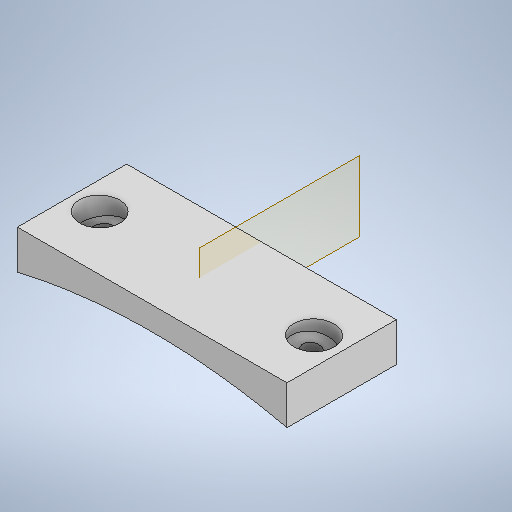
# Autodesk Inventor part: MountPlateV1
Saved by Autodesk Inventor 2025 (Build 290162000, 162)
## iProperties
Created: 2024-05-27
Part Number: MountPlateV1
Material: Generic
Document SubType Name: Modeling
Designer: mason
Density: 1 g/cm^3
Appearance: Default
Author: mason
Autodesk Inventor part; units mm, degrees
ref_plane "YZ Plane" through (0, 0, 0) normal (1, 0, 0) x (0, 1, 0)
ref_plane "XZ Plane" through (0, 0, 0) normal (0, 1, 0) x (-1, 0, 0)
ref_plane "XY Plane" through (0, 0, 0) normal (0, 0, 1) x (1, 0, 0)
sketch "Sketch3" plane through (0, 0, 0) normal (0, 0, 1) x (1, 0, 0)
  line L0 (11.505, 42.3202) -> (113.105, 42.3202)
  line L1 (113.105, 42.3202) -> (113.105, 16.9202)
  line L2 (113.105, 16.9202) -> (11.505, 16.9202)
  line L3 (11.505, 16.9202) -> (11.505, 42.3202)
  point P0 (0, 0)
  dimension "d11" = 101.6
  dimension "d12" = 25.4
  constraints: 8 end point, 2 parallel, 1 horizontal, 1 perpendicular
  measures "d11" distance of L1.end L2.end
  measures "d12" distance of L0.end L1.end
extrude "Extrusion1" add sketch "Sketch3" along normal blind 50.8
sketch "Sketch4" plane through (0, 0, 50.8) normal (0, 0, 1) x (1, 0, 0)
  line L0 (11.505, 16.9202) -> (113.105, 16.9202) projected
  line L1 (62.305, 23.2702) -> (62.305, 26.3182)
  line L2 (97.738, 23.2702) -> (26.872, 23.2702)
  circle A0 centre (62.305, -181.1601) radius 207.4783
  point P0 (0, 0)
  constraints: 4 end point, 3 point on circle, 1 centre point, 1 horizontal
extrude "Extrusion2" cut sketch "Sketch4" against normal blind 50.8
sketch "Sketch6" plane through (0, 0, 50.8) normal (0, 0, 1) x (1, 0, 0)
  arc A0 (113.105, 20.003) -> (11.505, 20.003) centre (62.305, -181.1601) ccw projected
  line L0 (62.305, 26.3182) -> (62.305, 23.2702)
  line L1 (62.305, 23.2702) -> (26.872, 23.2702)
  line L2 (26.872, 23.2702) -> (97.738, 23.2702)
  arc A1 (97.738, 23.2702) -> (26.872, 23.2702) centre (62.305, -181.1601) ccw
  line L3 (26.872, 23.2702) -> (29.8127, 23.7797)
  line L4 (26.872, 23.2702) -> (29.8565, 23.2702) construction
  line L5 (29.8127, 23.7797) -> (28.7286, 30.0365)
  line L6 (28.7286, 30.0365) -> (32.6703, 30.7195)
  line L7 (32.6703, 30.7195) -> (32.0199, 34.4735)
  line L8 (26.872, 23.2702) -> (22.5356, 48.2973)
  line L9 (26.872, 23.2702) -> (52.272, 23.2702) construction
  line L10 (22.5356, 48.2973) -> (29.418, 49.4898)
  line L11 (29.418, 49.4898) -> (32.0199, 34.4735)
  line L12 (29.8127, 23.7797) -> (29.9804, 22.8117)
  line L13 (29.9804, 22.8117) -> (27.0397, 22.3022)
  line L14 (27.0397, 22.3022) -> (26.872, 23.2702)
  point P0 (0, 0)
  dimension "d39" = 3.048
  dimension "d40" = 35.433
  dimension "d41" = 2.9845
  dimension "d42" = 9.83
  dimension "d43" = 6.35
  dimension "d44" = 90
  dimension "d45" = 4.0005
  dimension "d46" = 90
  dimension "d47" = 3.81
  dimension "d48" = 25.4
  dimension "d49" = 99.83
  constraints: 30 end point, 7 perpendicular, 6 point on circle, 2 equal length, 2 horizontal, 2 point on line, 1 centre point, 1 vertical
  measures "d39" distance of L0.start L0.end
  measures "d40" distance of L0.end L1.end
  measures "d41" distance of L1.end L3.end
  measures "d42" angle of L4 L3
  measures "d43" distance of L3.end L5.end
  measures "d44" angle of L5 L3
  measures "d45" distance of L5.end L6.end
  measures "d46" angle of L5 L6
  measures "d47" distance of L6.end L7.end
  measures "d48" distance of L1.end L8.end
  measures "d49" angle of L9 L8
revolve "Revolution1" cut sketch "Sketch6" angle 360 about axis through (26.872, 23.2702, 50.8) along (-0.1707254, 0.9853186, 0) contours L12 L1 A0 | A0 L3 L12 | L12 L13 L14 L1 | L8 L10 L11 L7 L6 L5 L3
ref_plane "Work Plane2" through (62.305, 42.3202, 50.8) normal (1, 0, 0) x (0, 0, -1)
mirror "Mirror1" about plane through (62.305, 42.3202, 50.8) normal (1, 0, 0) of "Revolution1"
sketch "Sketch7" plane through (0, 0, 50.8) normal (0, 0, 1) x (1, 0, 0)
  line L0 (18.9054, 28.3344) -> (16.4821, 42.3202) projected
  line L1 (18.9054, 28.3344) -> (18.255, 32.0885)
  line L2 (18.255, 32.0885) -> (32.0199, 34.4735)
  line L3 (32.0199, 34.4735) -> (32.6703, 30.7195)
  line L4 (32.0199, 34.4735) -> (113.105, 34.4735)
  line L5 (113.105, 20.003) -> (113.105, 42.3202) projected
  line L6 (16.4821, 42.3202) -> (11.505, 42.3202) projected
  line L7 (113.105, 34.4735) -> (11.505, 34.4735)
  line L8 (11.505, 34.4735) -> (11.505, 42.3202)
  line L9 (11.505, 42.3202) -> (113.105, 42.3202)
  line L10 (113.105, 42.3202) -> (113.105, 34.4735)
  point P0 (0, 0)
  dimension "d52" = 3.81
  dimension "d53" = 13.97
  dimension "d54" = 90
  constraints: 16 end point, 3 perpendicular, 2 horizontal, 2 parallel, 2 point on line
  measures "d52" distance of L0.start L1.end
  measures "d53" distance of L1.end L2.end
  measures "d54" angle of L1 L2
extrude "Extrusion3" cut sketch "Sketch7" against normal blind 50.8 contours L7 L8 L6 L0 | L0 L9 L5 L4 L7
sketch "Sketch8" plane through (0, 0, 50.8) normal (0, 0, 1) x (1, 0, 0)
  line L0 (18.9054, 28.3344) -> (17.8417, 34.4735) projected
  line L1 (17.8417, 34.4735) -> (15.3017, 34.4735)
  line L2 (11.505, 34.4735) -> (113.105, 34.4735) projected
  line L3 (15.3017, 34.4735) -> (15.3017, 16.7671)
  line L4 (15.3017, 16.7671) -> (7.6342, 16.7671)
  line L5 (7.6342, 16.7671) -> (7.6342, 34.4735)
  line L6 (7.6342, 34.4735) -> (15.3017, 34.4735)
  line L7 (62.305, 34.4735) -> (62.305, 19.3718)
  line L8 (109.3083, 34.4735) -> (109.3083, 16.7671)
  line L9 (109.3083, 16.7671) -> (116.9758, 16.7671)
  line L10 (116.9758, 16.7671) -> (116.9758, 34.4735)
  line L11 (116.9758, 34.4735) -> (109.3083, 34.4735)
  point P0 (0, 0)
  dimension "d57" = 2.54
  constraints: 20 end point, 4 perpendicular, 4 symmetric about line, 2 point on line, 1 midpoint, 1 vertical
  measures "d57" distance of L0.end L1.end
extrude "Extrusion4" cut sketch "Sketch8" against normal blind 50.8
sketch "Sketch9" plane through (0, 0, 0) normal (0, 0, -1) x (-1, 0, 0)
  line L0 (-123.5208, 45.9759) -> (-4.4224, 45.9759)
  line L1 (-4.4224, 45.9759) -> (-4.4224, 6.2764)
  line L2 (-4.4224, 6.2764) -> (-123.5208, 6.2764)
  line L3 (-123.5208, 6.2764) -> (-123.5208, 45.9759)
  point P0 (0, 0)
  constraints: 8 end point, 2 parallel, 1 horizontal, 1 perpendicular
extrude "Extrusion5" cut sketch "Sketch9" against normal blind 31.75
sketch "Sketch10" plane through (0, 0, 50.8) normal (0, 0, 1) x (1, 0, 0)
  arc A0 (23.935, 22.7393) -> (15.3017, 20.9239) centre (62.305, -181.1601) ccw projected
  line L0 (15.3017, 34.4735) -> (15.3017, 20.9239) projected
  line L1 (15.3017, 20.9239) -> (15.3017, 34.4735)
  line L2 (109.3083, 20.9239) -> (109.3083, 34.4735) projected
  line L3 (15.3017, 34.4735) -> (109.3083, 34.4735)
  line L4 (109.3083, 34.4735) -> (109.3083, 20.9239)
  arc A1 (109.3083, 20.9239) -> (15.3017, 20.9239) centre (62.305, -181.1601) ccw
  point P0 (0, 0)
  point P1 (23.935, 22.7393)
  constraints: 6 end point, 2 perpendicular, 2 point on circle, 1 centre point, 1 collinear
extrude "Extrusion6" add sketch "Sketch10" along normal blind 19.05
mirror "Mirror5" about plane through (62.305, 27.6987, 50.8) normal (0, 0, -1) of "Revolution1", "Mirror1"
body "Solid1"
